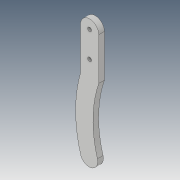
# Autodesk Inventor part: gripperPart5
Saved by Autodesk Inventor 2018 (Build 220112000, 112)
## iProperties
Created: 2020-01-20
Part Number: gripperPart5
Material: Generic
Document SubType Name: Modeling
Designer: anirudh
Density: 1 g/cm^3
Appearance: Default
Author: anirudh
Autodesk Inventor part; units mm, degrees
ref_plane "YZ Plane" through (0, 0, 0) normal (1, 0, 0) x (0, 1, 0)
ref_plane "XZ Plane" through (0, 0, 0) normal (0, 1, 0) x (-1, 0, 0)
ref_plane "XY Plane" through (0, 0, 0) normal (0, 0, 1) x (1, 0, 0)
sketch "Sketch1" plane through (0, 0, 0) normal (0, 0, 1) x (1, 0, 0)
  arc A0 (5.6515, 0) -> (-5.6515, 0) centre (0, 0) ccw
  line L0 (-5.6515, -38.1) -> (-5.6515, 0)
  line L1 (5.6515, -38.1) -> (5.6515, 0)
  line L2 (-5.6515, -38.1) -> (5.6515, -38.1)
  circle A1 centre (0, 0) radius 1.75
  circle A2 centre (0, -23.4188) radius 1.75
  dimension "d0" = 11.303
  dimension "d2" = 3.5
  dimension "d6" = 3.5
  constraints: 6 end point, 3 centre point, 2 coincident, 2 point on circle, 1 horizontal, 1 parallel, 1 vertical
  measures "d0" diameter of A0
  measures "d2" diameter of A1
  measures "d6" diameter of A2
extrude "Extrusion2" add sketch "Sketch1" along normal blind 5.08
sketch "Sketch2" plane through (0, 0, 5.08) normal (0, 0, 1) x (1, 0, 0)
  line L0 (-5.6515, 0) -> (-5.6515, -38.1) projected
  arc A0 (-5.6515, -38.1) -> (-5.6515, -101.6) centre (90.8601, -69.85) ccw
  line L1 (-5.6515, -38.1) -> (5.6515, -38.1) projected
  arc A1 (5.6515, -38.1) -> (4.7062, -98.5676) centre (102.1631, -69.85) ccw
  arc A2 (-5.6515, -101.6) -> (4.606, -98.2255) centre (-0.5227, -99.9128) ccw
  line L2 (-5.6515, -38.1) -> (5.6515, -38.1)
  point P0 (0, 0)
  dimension "d11" = 63.5
  dimension "d12" = 101.6
  dimension "d13" = 101.6
  constraints: 8 point on circle, 3 centre point, 2 end point, 1 collinear, 1 point on line
  measures "d11" distance of L0.end A0.end
  measures "d12" radius of A0
  measures "d13" radius of A1
extrude "Extrusion3" add sketch "Sketch2" against normal blind 5.08 contours L1 A1 A2 A0
sketch "Sketch3" plane through (0, 0, 5.08) normal (0, 0, 1) x (1, 0, 0)
  arc A0 (8.255, 0) -> (-8.255, 0) centre (0, 0) ccw
  line L0 (-8.255, 0) -> (-8.255, -38.1)
  line L1 (8.255, 0) -> (8.255, -38.1)
  arc A1 (-8.255, -101.3562) -> (7.0262, -97.7027) centre (-0.5227, -99.9128) ccw
  arc A2 (8.255, -38.1) -> (7.0262, -97.7027) centre (102.1631, -69.85) ccw
  arc A3 (-8.255, -38.3438) -> (-7.8126, -102.8673) centre (102.1631, -69.85) ccw
  line L2 (-8.255, -35.1418) -> (-8.255, -38.3438)
  circle A4 centre (0, 0) radius 1.75
  circle A5 centre (0, -23.4188) radius 1.75 projected
  circle A6 centre (0, -23.4188) radius 1.75
  dimension "d18" = 16.51
  constraints: 10 point on circle, 6 centre point, 6 coincident, 6 end point, 3 vertical, 2 point on line
  measures "d18" diameter of A0
extrude "Extrusion4" add sketch "Sketch3" against normal blind 5.08 contours L1 A2 A1 A3 L2 L0 A0
body "Solid2"
